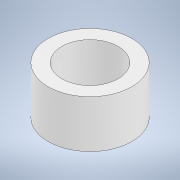
# Autodesk Inventor part: knobBushing
Saved by Autodesk Inventor 2022.2 (Build 262287000, 287)
## iProperties
Created: 2021-12-28
Part Number: knobBushing
Material: PC/ABS Plastic
Document SubType Name: Modeling
Designer: robst
Density: 0.357273 g/cm^3
Appearance: Smooth - White
Author: robst
Autodesk Inventor part; units mm, degrees
ref_plane "YZ Plane" through (0, 0, 0) normal (1, 0, 0) x (0, 1, 0)
ref_plane "XZ Plane" through (0, 0, 0) normal (0, 1, 0) x (-1, 0, 0)
ref_plane "XY Plane" through (0, 0, 0) normal (0, 0, 1) x (1, 0, 0)
sketch "Sketch1" plane through (0, 0, 0) normal (0, 1, 0) x (-1, 0, 0)
  circle A0 centre (0, 0) radius 9.398
  circle A1 centre (0, 0) radius 13.97
  dimension "d0" = 18.796
  dimension "d1" = 27.94
  constraints: 2 centre point, 2 coincident
  measures "d0" diameter of A0
  measures "d1" diameter of A1
extrude "Extrusion1" add sketch "Sketch1" against normal blind 15.875
equation "\"d0\" = insideDiameter"
equation "\"d1\" = outsideDiameter"
equation "\"d2\" = height"
equation "\"insideDiameter\" = 18.796"
equation "\"outsideDiameter\" = 27.94"
equation "\"height\" = 15.875"
body "Solid1"
